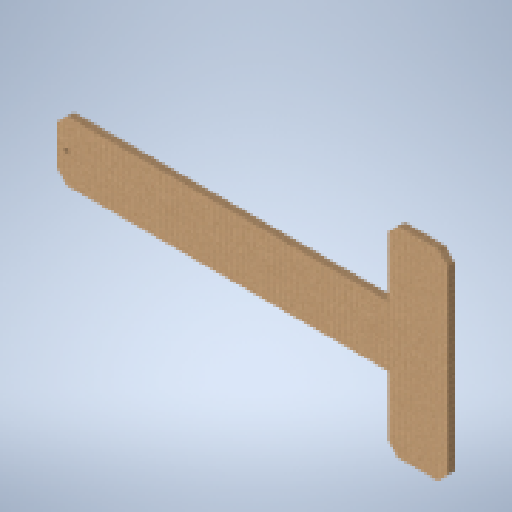
# Autodesk Inventor part: PistonV2
Saved by Autodesk Inventor 2023.1 (Build 271208000, 208)
## iProperties
Created: 2022-10-30
Part Number: PistonV2
Material: MDF Medium Density Fiberboard
Document SubType Name: Modeling
Designer: Daniel Peña
Density: 0.8 g/cm^3
Appearance: Cardboard - Corrugated
Author: Daniel Peña
Autodesk Inventor part; units mm, degrees
ref_plane "YZ Plane" through (0, 0, 0) normal (1, 0, 0) x (0, 1, 0)
ref_plane "XZ Plane" through (0, 0, 0) normal (0, 1, 0) x (-1, 0, 0)
ref_plane "XY Plane" through (0, 0, 0) normal (0, 0, 1) x (1, 0, 0)
sketch "Sketch1" plane through (0, 0, 0) normal (0, 0, 1) x (1, 0, 0)
  line L0 (115.5719, 99.9144) -> (75.5719, 99.9144)
  line L1 (75.5719, -100.0856) -> (115.5719, -100.0856)
  line L2 (125.5719, -90.0856) -> (125.5719, 89.9144)
  line L3 (65.5719, 29.9144) -> (-254.4281, 29.9144)
  line L4 (-264.4281, 19.9144) -> (-264.4281, -20.0856)
  line L5 (-254.4281, -30.0856) -> (65.5719, -30.0856)
  line L6 (65.5719, 89.9144) -> (65.5719, 29.9144)
  line L7 (65.5719, -30.0856) -> (65.5719, -90.0856)
  line L8 (125.5719, -0.0856) -> (-264.4281, -0.0856) construction
  line L9 (125.5719, 89.9144) -> (115.5719, 99.9144)
  line L10 (75.5719, 99.9144) -> (65.5719, 89.9144)
  line L11 (115.5719, -100.0856) -> (125.5719, -90.0856)
  line L12 (75.5719, -100.0856) -> (65.5719, -90.0856)
  line L13 (-254.4281, -30.0856) -> (-264.4281, -20.0856)
  line L14 (-264.4281, 19.9144) -> (-254.4281, 29.9144)
  point P0 (0, 0)
  point P1 (125.5719, 99.9144)
  point P2 (65.5719, -100.0856)
  point P3 (65.5719, 99.9144)
  point P4 (125.5719, -100.0856)
  point P5 (-264.4281, -30.0856)
  point P6 (-264.4281, 29.9144)
  dimension "d0" = 60
  dimension "d2" = 330
  dimension "d3" = 60
  dimension "d4" = 200
  dimension "d5" = 10
  dimension "d6" = 10
  dimension "d7" = 10
  dimension "d8" = 10
  dimension "d9" = 10
  dimension "d10" = 10
  dimension "d11" = 10
  dimension "d12" = 10
  dimension "d13" = 10
  dimension "d14" = 10
  dimension "d15" = 10
  dimension "d16" = 10
  constraints: 30 end point, 12 point on line, 4 parallel, 4 perpendicular, 2 horizontal, 2 midpoint, 1 collinear, 1 other
  measures "d0" distance of point (125.572, -100.086) point (65.572, -100.086)
  measures "d2" distance of L5.end point (-264.428, -30.086)
  measures "d3" distance of point (-264.428, -30.086) point (-264.428, 29.914)
  measures "d4" distance between parallel lines of L1 L0
  measures "d5" distance of L2.end point (125.572, 99.914)
  measures "d6" distance of L0.start point (125.572, 99.914)
  measures "d7" distance of L0.end point (65.572, 99.914)
  measures "d8" distance of L6.start point (65.572, 99.914)
  measures "d9" distance of L1.end point (125.572, -100.086)
  measures "d10" distance of L2.start point (125.572, -100.086)
  measures "d11" distance of L1.start point (65.572, -100.086)
  measures "d12" distance of L7.end point (65.572, -100.086)
  measures "d13" distance of L5.start point (-264.428, -30.086)
  measures "d14" distance of L4.end point (-264.428, -30.086)
  measures "d15" distance of L4.start point (-264.428, 29.914)
  measures "d16" distance of L3.end point (-264.428, 29.914)
extrude "Extrusion1" add sketch "Sketch1" along normal blind 7
sketch "Sketch2" plane through (0, 0, 7) normal (0, 0, 1) x (1, 0, 0)
  line L0 (-264.4281, 19.9144) -> (-264.4281, -20.0856) projected
  point P0 (0, 0)
  point P1 (-254.4281, 0)
  dimension "d19" = 10
  measures "d19" distance from line of L0 point (-254.428, 0)
hole "Hole1" at (-254.4281, 0, 7) direction (0, 0, -1) diameter 5 end through all
equation "\"d6\" = d5"
equation "\"d7\" = d5"
equation "\"d8\" = d7"
equation "\"d9\" = d5"
equation "\"d10\" = d9"
equation "\"d11\" = d5"
equation "\"d12\" = d11"
equation "\"d13\" = d5"
equation "\"d14\" = d13"
equation "\"d15\" = d5"
equation "\"d16\" = d15"
body "Solid1"
